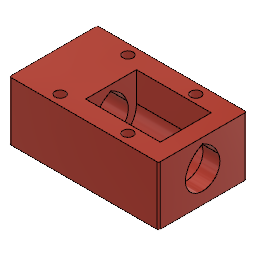
Carriage v2 (Autodesk Fusion 360 design; units mm, degrees)
Autodesk Fusion 360 part; units mm, degrees
sketch "Sketch1" plane through (0, 0, 0) normal (0, 1, 0) x (1, 0, 0)
  line L0 (-21.53, 13) -> (22.5, 13)
  line L1 (22.5, 13) -> (22.5, -13)
  line L2 (22.5, -13) -> (-21.53, -13)
  line L3 (-21.53, -13) -> (-21.53, 13)
  line L4 (-9.515, 10) -> (10.485, 10) construction
  line L5 (10.485, 10) -> (10.485, -10) construction
  line L6 (10.485, -10) -> (-9.515, -10) construction
  line L7 (-9.515, -10) -> (-9.515, 10) construction
  circle A0 centre (-9.515, 10) radius 1.5
  circle A1 centre (10.485, 10) radius 1.5
  circle A2 centre (-9.515, -10) radius 1.5
  circle A3 centre (10.485, -10) radius 1.5
  dimension "d1" = 44.03
  dimension "d2" = 26
  dimension "d3" = 13
  dimension "d4" = 22.5
  dimension "d5" = 20
  dimension "d6" = 20
  dimension "d7" = 10
  dimension "d9" = 3
  dimension "d21" = 12.015
  dimension "d22" = 12.015
  measures "d3" distance of origin
  measures "d4" distance of origin
  measures "d7" distance of origin
  measures "d9" diameter of A0
  measures "d21" distance of L1
  measures "d22" distance of L3
extrude "Extrude1" add sketch "Sketch1" along normal blind 17.3
sketch "Sketch2" plane through (22.5, 0, 0) normal (1, 0, 0) x (0, 0, -1)
  line L0 (-13, 0) -> (13, 0)
  line L1 (13, 0) -> (13, 17.3)
  line L2 (13, 17.3) -> (-13, 17.3)
  line L3 (-13, 17.3) -> (-13, 0)
  circle A0 centre (0, 8.65) radius 5.1
  line L4 (0, 8.65) -> (0, 15.65) construction
  spline S0 degree 5 poles (-5.1, 8.65) (-5.0352, 9.1709) (-4.8649, 10.1424) (-4.4878, 11.3888) (-3.775, 12.6875) (-2.6511, 13.9078) (-1.6378, 14.6862) (-0.8346, 15.1953) (-0.2812, 15.5036) (0, 15.65) knots 0 0 0 0 0 0 0.2 0.4 0.6 0.8 1 1 1 1 1 1
  spline S1 degree 5 poles (5.1, 8.65) (5.0352, 9.1709) (4.8649, 10.1424) (4.4878, 11.3888) (3.775, 12.6875) (2.6511, 13.9078) (1.6378, 14.6862) (0.8346, 15.1953) (0.2812, 15.5036) (0, 15.65) knots 0 0 0 0 0 0 0.2 0.4 0.6 0.8 1 1 1 1 1 1
  line L5 (-5.2556, 7.4) -> (-4.9444, 9.9)
  line L6 (5.2556, 7.4) -> (4.9444, 9.9)
  dimension "d12" = 10.2
  dimension "d13" = 8.65
  dimension "d39" = 7
  dimension "d40" = 1.25
  dimension "d41" = 1.25
  measures "d12" diameter of A0
  measures "d13" distance of origin
extrude "Extrude2" cut sketch "Sketch2" against normal through all contours A0 L6 | A0 S0 S1 | A0 S1 L6 | A0 S0 L5 | A0 L5 | A0 S0 S1
sketch "Sketch3" plane through (22.5, 0, 0) normal (1, 0, 0) x (0, 0, -1)
  line L0 (-13, 0) -> (13, 0)
  line L1 (13, 0) -> (13, 17.3)
  line L2 (13, 17.3) -> (-13, 17.3)
  line L3 (-13, 17.3) -> (-13, 0)
  circle A0 centre (0, 8.65) radius 8 construction
  circle A1 centre (-8, 8.65) radius 2.1
  circle A2 centre (0, 16.65) radius 2.1 construction
  circle A3 centre (8, 8.65) radius 2.1
  arc A4 (-4.6029, 10.8463) -> (4.6029, 10.8463) centre (0, 8.65) ccw
  spline S0 degree 5 poles (-4.6029, 10.8463) (-4.5981, 10.8597) (-4.4535, 11.2644) (-4.1328, 11.9971) (-3.5579, 12.9232) (-2.6511, 13.9078) (-1.6378, 14.6862) (-0.8346, 15.1953) (-0.2812, 15.5036) (0, 15.65) knots 0.193129 0.193129 0.193129 0.193129 0.193129 0.193129 0.2 0.4 0.6 0.8 1 1 1 1 1 1
  spline S1 degree 5 poles (0, 15.65) (0.2812, 15.5036) (0.8346, 15.1953) (1.6378, 14.6862) (2.6511, 13.9078) (3.5579, 12.9232) (4.1328, 11.9971) (4.4535, 11.2644) (4.5981, 10.8597) (4.6029, 10.8463) knots -1 -1 -1 -1 -1 -1 -0.8 -0.6 -0.4 -0.2 -0.193129 -0.193129 -0.193129 -0.193129 -0.193129 -0.193129
  dimension "d15" = 16
  dimension "d16" = 4.2
  dimension "d17" = 4.2
  dimension "d18" = 4.2
  measures "d15" diameter of A0
  measures "d16" diameter of A1
  measures "d17" diameter of A2
  measures "d18" diameter of A3
fillet "Fillet2" radius 0.5 curvature continuous 4 edges at (-21.53, 8.65, 13) (22.5, 8.65, 13) (22.5, 8.65, -13) (-21.53, 8.65, -13)
sketch "Sketch9" plane through (22.5, 0, 0) normal (1, 0, 0) x (0, 0, -1)
  arc A0 (-4.6029, 10.8463) -> (4.6029, 10.8463) centre (0, 8.65) ccw
  spline S0 degree 5 poles (-4.6029, 10.8463) (-4.5981, 10.8597) (-4.4535, 11.2644) (-4.1328, 11.9971) (-3.5579, 12.9232) (-2.6511, 13.9078) (-1.6378, 14.6862) (-0.8346, 15.1953) (-0.2812, 15.5036) (0, 15.65) knots 0.193129 0.193129 0.193129 0.193129 0.193129 0.193129 0.2 0.4 0.6 0.8 1 1 1 1 1 1
  spline S1 degree 5 poles (0, 15.65) (0.2812, 15.5036) (0.8346, 15.1953) (1.6378, 14.6862) (2.6511, 13.9078) (3.5579, 12.9232) (4.1328, 11.9971) (4.4535, 11.2644) (4.5981, 10.8597) (4.6029, 10.8463) knots -1 -1 -1 -1 -1 -1 -0.8 -0.6 -0.4 -0.2 -0.193129 -0.193129 -0.193129 -0.193129 -0.193129 -0.193129
  line L0 (12.5, 0) -> (12.5, 17.3)
  line L1 (12.5, 17.3) -> (-12.5, 17.3)
  line L2 (-12.5, 17.3) -> (-12.5, 0)
  line L3 (-12.5, 0) -> (12.5, 0)
  circle A1 centre (0, 8.65) radius 7.5
  line L4 (-7.5, 8.65) -> (7.5, 8.65)
  line L5 (7.5, 8.65) -> (7.5, 17.3)
  line L6 (7.5, 17.3) -> (-7.5, 17.3)
  line L7 (-7.5, 17.3) -> (-7.5, 8.65)
  dimension "d45" = 15
  measures "d45" diameter of A1
extrude "Extrude7" cut sketch "Sketch9" against normal blind 22 from surface at -5 contours A0 S0 S1 A1 L4 | A0 A1 L4 | L1 A1 L5 L6 L7
equation "d1 = 45 mm - ( ( 0.485 * 2 ) * 1 mm )"
equation "d4 = ( 45 / 2 ) * 1 mm"
equation "d10 = ( 8.65 * 2 ) * 1 mm"
equation "d21 = 12.50 mm - 0.485 mm"
